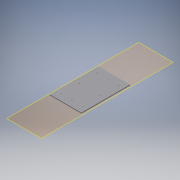
# Autodesk Inventor part: components_board
Saved by Autodesk Inventor 2017 SP1 (Build 210196100, 196)
## iProperties
Part Number: components_board
Material: 一般
Document SubType Name: Modeling
Designer: gisen
Density: 1 g/cm^3
Appearance: 既定
Author: gisen
Autodesk Inventor part; units mm, degrees
ref_plane "YZ Plane" through (0, 0, 0) normal (1, 0, 0) x (0, 1, 0)
ref_plane "XZ Plane" through (0, 0, 0) normal (0, 1, 0) x (-1, 0, 0)
ref_plane "XY Plane" through (0, 0, 0) normal (0, 0, 1) x (1, 0, 0)
ref_plane "作業平面1" through (0, 0, 0) normal (0, 0, 1) x (1, 0, 0)
sketch "スケッチ1" plane through (0, 0, 0) normal (0, 0, 1) x (1, 0, 0)
  line L0 (0, -891.1557) -> (0, 228.8443)
  line L1 (-147, -331.1557) -> (147, -331.1557)
  circle A0 centre (72, -331.1557) radius 2.25 projected
  circle A1 centre (-72, -211.1557) radius 2.25 projected
  circle A2 centre (0, -451.1557) radius 2.25 projected
  circle A3 centre (-72, -331.1557) radius 2.25 projected
  circle A4 centre (0, -331.1557) radius 2.25 projected
  circle A5 centre (-72, -451.1557) radius 2.25 projected
  circle A6 centre (0, -211.1557) radius 2.25 projected
  circle A7 centre (72, -451.1557) radius 2.25 projected
  circle A8 centre (72, -211.1557) radius 2.25 projected
  circle A9 centre (20.5, -135.3359) radius 2.75 projected
  circle A10 centre (20.5, -72.3359) radius 2.75 projected
  circle A11 centre (-20.5, -585.3359) radius 2.75 projected
  circle A12 centre (20.5, -522.3359) radius 2.75 projected
  circle A13 centre (-20.5, -522.3359) radius 2.75 projected
  circle A14 centre (20.5, -585.3359) radius 2.75 projected
  circle A15 centre (-20.5, -72.3359) radius 2.75 projected
  circle A16 centre (-20.5, -135.3359) radius 2.75 projected
  arc A17 (105, -36.1557) -> (-105, -36.1557) centre (0, -36.1557) ccw projected
  line L2 (-105, -626.1557) -> (-105, -36.1557) projected
  arc A18 (-105, -626.1557) -> (105, -626.1557) centre (0, -626.1557) ccw projected
  line L3 (105, -36.1557) -> (105, -626.1557) projected
  line L4 (105, -493.6557) -> (-105, -493.6557)
  line L5 (-105, -493.6557) -> (-105, -168.6557)
  line L6 (-105, -168.6557) -> (105, -168.6557)
  line L7 (105, -168.6557) -> (105, -493.6557)
  line L8 (105, -493.6557) -> (-105, -168.6557) construction
  line L9 (-105, -493.6557) -> (105, -168.6557) construction
  point P0 (0, 0)
  dimension "d0" = 325
  constraints: 16 end point, 2 horizontal, 2 midpoint, 2 parallel, 1 perpendicular, 1 point on line, 1 vertical, 4 other
  measures "d0" distance of L4.end L5.end
extrude "押し出し1" add sketch "スケッチ1" along normal blind 5 contours L4 L2 L1 A3 A4 L0 A2 | L0 A2 A4 L1 A0 L3 L4 | L1 A0 A4 L0 A6 L6 L3 | L2 L6 L0 A6 A4 L1 A3
